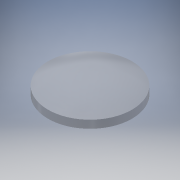
# Autodesk Inventor part: 00_CollectorLens-30mm
Saved by Autodesk Inventor 2016 (Build 200138000, 138)
## iProperties
Created: 2016-09-10
Part Number: 00_CollectorLens-30mm
Material: Generisch
Document SubType Name: Modeling
Designer: Bene
Density: 1 g/cm^3
Appearance: Polycarbonat - klar
Mass: 1.34537 g
Surface Area: 8.79172 cm^2
Volume: 1.34537 cm^3
Author: Bene
Autodesk Inventor part; units mm, degrees
ref_plane "YZ Plane" through (0, 0, 0) normal (1, 0, 0) x (0, 1, 0)
ref_plane "XZ Plane" through (0, 0, 0) normal (0, 1, 0) x (-1, 0, 0)
ref_plane "XY Plane" through (0, 0, 0) normal (0, 0, 1) x (1, 0, 0)
sketch "Skizze1" plane through (0, 0, 0) normal (0, 1, 0) x (-1, 0, 0)
  arc A0 (0, 0) -> (21.5, 0) centre (10.75, 33.3082) ccw
  line L0 (0, 0) -> (21.5, 0)
  line L1 (21.5, 0) -> (21.5, 2)
  line L2 (21.5, 2) -> (0, 2)
  line L3 (0, 2) -> (0, 0)
  arc A1 (21.5, 2) -> (0, 2) centre (10.75, -31.3082) ccw
  line L4 (10.75, -1.6918) -> (10.75, 3.6918)
  point P0 (10.75, 0)
  point P1 (10.75, 2)
  point P2 (0.0868, 2.1341)
  dimension "d0" = 21.5
  dimension "d1" = 35
  dimension "d2" = 2
  dimension "d3" = 35
  constraints: 10 end point, 6 point on circle, 4 coincident, 2 centre point, 2 midpoint, 2 parallel, 2 point on line, 1 horizontal, 1 perpendicular
  measures "d0" distance of L0.start A0.end
  measures "d1" radius of A0
  measures "d2" distance of L1.end L0.end
  measures "d3" radius of A1
revolve "Umdrehung1" add sketch "Skizze1" angle 360 about axis through (-10.75, 0, -1.6918) along (0, 0, 1) picked at (4.756, -0.3122) picked at (4.756, 2.3122) contours L0 L4 A0 | L3 L2 L4 L0 | A1 L4 L2
